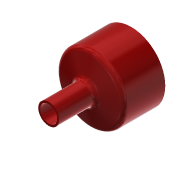
# Autodesk Inventor part: 01_Connector_T
Saved by Autodesk Inventor 2019.4 (Build 234330000, 330)
## iProperties
Created: 2021-06-01
Part Number: 01_Connector_T
Material: Generic
Document SubType Name: Modeling
Designer: diederichbenedict
Density: 1 g/cm^3
Appearance: Smooth - Red
Author: diederichbenedict
Autodesk Inventor part; units mm, degrees
ref_plane "YZ Plane" through (0, 0, 0) normal (1, 0, 0) x (0, 1, 0)
ref_plane "XZ Plane" through (0, 0, 0) normal (0, 1, 0) x (-1, 0, 0)
ref_plane "XY Plane" through (0, 0, 0) normal (0, 0, 1) x (1, 0, 0)
sketch "Sketch1" plane through (0, 0, 0) normal (1, 0, 0) x (0, 1, 0)
  line L0 (-11, 0) -> (11, 0)
  line L1 (13, -8.587477) -> (0, -8.587477)
  line L2 (0, -8.587477) -> (0, 9)
  line L3 (0, 9) -> (4, 9)
  line L4 (4, 9) -> (11, 0) construction
  line L5 (4, 9) -> (13, 7)
  line L6 (13, 7) -> (13, 2)
  line L7 (13, 2) -> (13, 0)
  line L8 (4, 9) -> (0, 9)
  line L9 (0, 9) -> (0, 23)
  line L10 (0, 23) -> (4, 23)
  line L11 (4, 23) -> (4, 9)
  line L12 (13, -8.587477) -> (13, 0)
  point P0 (0, 0)
  dimension "d12" = 4
  dimension "d13" = 0
  dimension "d15" = 13
  dimension "d16" = 0
  dimension "d17" = 2
  dimension "d19" = 5
  dimension "d20" = 14
  constraints: 24 end point, 4 parallel, 3 perpendicular, 2 horizontal, 2 point on line, 1 other
  measures "d12" distance between parallel lines of L11 L9
  measures "d13" distance from line of point (0, 0) L2
  measures "d15" distance of L1.end L1.start
  measures "d16" angle of L2 L12
  measures "d17" distance from line of L5.end L3
  measures "d19" distance of L6.end L5.end
  measures "d20" distance between parallel lines of L3 L10
revolve "Revolution1" add sketch "Sketch1" angle 360 about axis through (0, 0, -8.587477) along (0, 0, 1)
sketch "Sketch4" plane through (0, 0, 23) normal (0, 0, 1) x (1, 0, 0)
  circle A0 centre (0, 0) radius 1.479649
  circle A1 centre (0, 0) radius 4
  circle A2 centre (0, 0) radius 3.25
  point P0 (0, 0)
  dimension "d21" = 6.5
  constraints: 1 centre point, 1 coincident
  measures "d21" diameter of A2
extrude "Extrusion2" cut sketch "Sketch4" against normal through all contours A0 | A2
sketch "Sketch5" plane through (0, 0, -8.587477) normal (0, 0, -1) x (-1, 0, 0)
  circle A0 centre (0, 0) radius 11.938351
  circle A1 centre (0, 0) radius 11.2
  circle A2 centre (0, 0) radius 11
  point P0 (0, 0)
  dimension "d28" = 0.2
  constraints: 1 centre point
  measures "d28" radial gap between concentric circles of A2 A1
sketch "Sketch5 outline for Extrusion3" plane through (0, 0, -8.587477) normal (0, 0, -1) x (-1, 0, 0)
  circle A0 centre (0, 0) radius 11.2
extrude "Extrusion3" cut sketch "Sketch5 outline for Extrusion3" against normal blind 12 draft -3
fillet "Fillet2" radius 2 4 edges at (0, -4, 9) (0, -13, 7) (10.5711, 0, 3.4125) (-3.25, 0, 3.4125)
body "Solid1"
